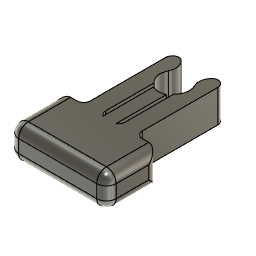
Fuse Holder v16 (Autodesk Fusion 360 design; units mm, degrees)
Autodesk Fusion 360 part; units mm, degrees
sketch "Sketch2" plane through (0, 0, 0) normal (0, 0, 1) x (1, 0, 0)
  line L0 (0, 0) -> (15, 0)
  line L1 (15, 0) -> (15, 8)
  line L2 (15, 8) -> (0, 8)
  line L3 (0, 8) -> (0, 0)
  line L4 (7.5, 8) -> (7.5, 18)
  circle A0 centre (7.5, 18) radius 2.25
  line L5 (7.5, 8) -> (6, 8)
  line L6 (6, 8) -> (6, 16.3229)
  line L7 (6, 8) -> (3.5, 8)
  line L8 (3.5, 8) -> (3.5, 20.6247)
  line L9 (7.5, 18) -> (7.4607, 20.2497)
  line L10 (7.5, 18) -> (9.75, 18) construction
  line L11 (4.9508, 21.5173) -> (7.4607, 20.2497)
  arc A1 (4.9508, 21.5173) -> (3.5, 20.6247) centre (4.5, 20.6247) ccw
  line L12 (9, 8) -> (9, 16.3229)
  line L13 (11.5, 8) -> (11.5, 20.6247)
  arc A2 (11.5, 20.6247) -> (10.0492, 21.5173) centre (10.5, 20.6247) ccw
  line L14 (10.0492, 21.5173) -> (7.5393, 20.2497)
  arc A3 (6.5, 15.7087) -> (7.5, 15.5) centre (7.5, 18) ccw
  line L15 (6.5, 8) -> (6.5, 15.7087)
  arc A4 (7.5, 15.5) -> (8.5, 15.7087) centre (7.5, 18) ccw
  line L16 (8.5, 8) -> (8.5, 15.7087)
  point P0 (3.5, 22.25)
  dimension "d24" = 15
  dimension "d25" = 8
  dimension "d26" = 10
  dimension "d27" = 4.5
  dimension "d28" = 1.5
  dimension "d29" = 2.5
  dimension "d30" = 14.25
  dimension "d31" = 91
  dimension "d32" = 1
  dimension "d37" = 5
  constraint horizontal L0
  constraint vertical L1
  constraint horizontal L2
  constraint vertical L3
  constraint coincident L0.start L3.end
  constraint midpoint L2 L4.start
  constraint perpendicular L2 L4
  constraint coincident L4.end A0.centre
  constraint perpendicular L4 L5
  constraint coincident A0 L6.end
  constraint perpendicular L2 L6
  constraint perpendicular L6 L7
  constraint vertical L8
  constraint horizontal L10
  constraint coincident A0 L9.end
  constraint coincident P0 L11
  constraint coincident P0 L8
  constraint tangent L11 A1
  constraint tangent L8 A1
  constraint symmetric L4 L5.end L12.start
  constraint symmetric L4 L6.end L12.end
  constraint symmetric L4 L7.end L13.start
  constraint symmetric L4 L9.end L14.end
  constraint symmetric L4 L11.start A2.end
  constraint symmetric L4 L8.end L13.end
  constraint symmetric L4 A1 A2
  constraint concentric A0 A3
  constraint coincident L4 A3.end
  constraint symmetric L4 A3 A4
  constraint symmetric L4 L15.start L16.start
  constraint symmetric L4 A3.start A4.end
  constraint symmetric L4 A3.end A4.start
  measures "d24" distance of L0.start L0.end
  measures "d25" distance of L0.start L2.end
  measures "d26" distance of L4.start L4.end
  measures "d27" diameter of A0
  measures "d28" distance of L4.start L5.end
  measures "d29" distance of L5.end L7.end
  measures "d30" distance of L7.end P0
  measures "d31" angle of L9 L10
  measures "d32" radius of A1
  measures "d37" diameter of A3
extrude "Extrude5" add sketch "Sketch2" along normal blind 5 contours L0 L1 L2 L3 L5 L7 | L2 A0 L6 L7 L8 L11 A1 | L2 A0 L12 L13 A2 L14 | L2 L4 L5 A3 L15 | L2 L4 A4 L16
fillet "Fillet4" radius 2 2 edges at (7.4607, 20.2497, 2.5) (7.5393, 20.2497, 2.5)
fillet "Fillet5" radius 1 2 edges at (6, 8, 2.5) (9, 8, 2.5)
fillet "Fillet6" radius 1 2 edges at (11.5, 8, 2.5) (3.5, 8, 2.5)
fillet "Fillet7" radius 1.5 10 edges at (0, 4, 5) (15, 4, 5) (15, 4, 0) (0, 4, 0) (0, 8, 2.5) (0, 0, 2.5) (7.5, 0, 5) (15, 0, 2.5) (7.5, 0, 0) (15, 8, 2.5)
equation "d30 = d26 + d27 / 2 + 2 mm"
